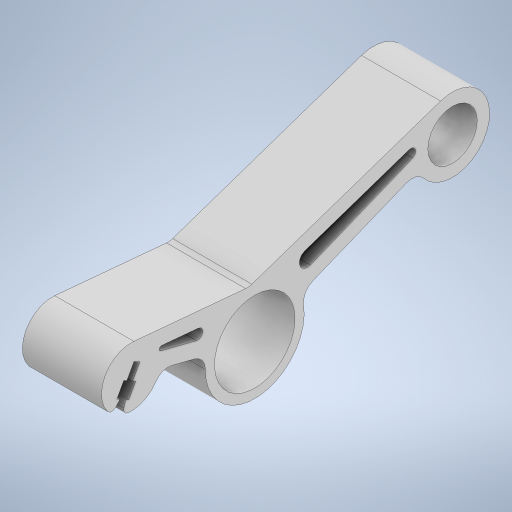
# Autodesk Inventor part: ChargingArm
Saved by Autodesk Inventor 2023 (Build 270158000, 158)
## iProperties
Created: 2023-03-28
Part Number: ChargingArm
Material: Generic
Document SubType Name: Modeling
Designer: ethan
Density: 1 g/cm^3
Appearance: Default
Author: ethan
Autodesk Inventor part; units mm, degrees
ref_plane "YZ Plane" through (0, 0, 0) normal (1, 0, 0) x (0, 1, 0)
ref_plane "XZ Plane" through (0, 0, 0) normal (0, 1, 0) x (-1, 0, 0)
ref_plane "XY Plane" through (0, 0, 0) normal (0, 0, 1) x (1, 0, 0)
sketch "Sketch1" plane through (0, 0, 0) normal (1, 0, 0) x (0, 1, 0)
  circle A0 centre (0, 0) radius 10
  circle A1 centre (0, 0) radius 8.15
  circle A2 centre (0, 0) radius 12.5 construction
  line L0 (41.321287, 101.306893) -> (-14.257578, 0) construction
  line L1 (-14.257578, 0) -> (54.700579, -125.694122) construction
  line L2 (0, 0) -> (-14.257578, 0) construction
  circle A3 centre (16.24172, -40) radius 7.5
  line L3 (23.342454, -37.585547) -> (9.467645, 3.219271)
  line L4 (0, 0) -> (16.24172, -40)
  circle A4 centre (6.301529, 25) radius 6
  line L5 (6.301529, 25) -> (0, 0)
  line L6 (12.276626, 24.45391) -> (9.958495, -0.91015)
  line L7 (6.301529, 25) -> (1.041169, 27.885933) construction
  line L8 (2.571626, 25.477961) -> (5.114134, 24.083094)
  line L9 (5.114134, 24.083094) -> (6.436853, 26.494093)
  line L10 (6.436853, 26.494093) -> (3.894345, 27.88896)
  line L11 (3.894345, 27.88896) -> (2.571626, 25.477961)
  line L12 (2.571626, 25.477961) -> (6.436853, 26.494093) construction
  line L13 (5.114134, 24.083094) -> (3.894345, 27.88896) construction
  line L14 (3.557653, 27.275251) -> (6.100161, 25.880384) construction
  line L15 (6.100161, 25.880384) -> (5.450826, 24.696803) construction
  line L16 (5.450826, 24.696803) -> (2.908318, 26.09167) construction
  line L17 (2.908318, 26.09167) -> (3.557653, 27.275251) construction
  line L18 (3.557653, 27.275251) -> (5.450826, 24.696803) construction
  line L19 (6.100161, 25.880384) -> (2.908318, 26.09167) construction
  line L20 (1.041169, 27.885933) -> (1.720669, 28.875012) construction
  line L21 (1.041169, 27.885933) -> (0.572083, 26.781415) construction
  line L22 (1.720669, 28.875012) -> (3.557653, 27.275251)
  line L23 (0.572083, 26.781415) -> (2.908318, 26.09167)
  circle A5 centre (16.24172, -40) radius 5
  line L24 (6.100161, 25.880384) -> (5.450826, 24.696803)
  line L25 (5.450826, 24.696803) -> (8.081006, 23.253836)
  line L26 (8.081006, 23.253836) -> (8.730341, 24.437418)
  line L27 (8.730341, 24.437418) -> (6.100161, 25.880384)
  line L28 (7.879427, 18.985837) -> (6.064574, 11.785787)
  line L29 (8.750781, 18.837133) -> (8.074972, 11.442697)
  circle A6 centre (8.309301, 18.877482) radius 0.44332
  circle A7 centre (7.056384, 11.53579) radius 1.022833
  line L30 (10.828915, -10.103009) -> (18.023548, -31.261908)
  line L31 (7.742377, -11.093657) -> (16.206515, -31.939079)
  circle A8 centre (9.297434, -10.623756) radius 1.617595
  circle A9 centre (17.10522, -31.574166) radius 0.969965
  point P0 (3.762124, -9.265334)
  point P1 (13.420127, -33.050999)
  point P2 (10.151966, 1.206731)
  point P3 (4.835032, 19.181978)
  point P4 (2.444163, 9.696704)
  point P5 (4.504239, 25.986027)
  point P6 (3.557653, 27.275251)
  point P7 (3.228968, 26.676138)
  point P8 (6.100161, 25.880384)
  point P9 (5.450826, 24.696803)
  point P10 (7.798679, -11.232315)
  dimension "d8" = 15
  dimension "d0" = 20
  dimension "d1" = 16.3
  dimension "d6" = 25
  dimension "d7" = 122.5
  dimension "d9" = 40
  dimension "d10" = 12
  dimension "d11" = 25
  dimension "d14" = 2.9
  dimension "d15" = 2.75
  dimension "d16" = 2.5
  dimension "d17" = 1.35
  dimension "d18" = 1.2
  dimension "d19" = 1.2
  dimension "d20" = 10
  dimension "d24" = 3
  dimension "d25" = 3
  dimension "d26" = 3
  dimension "d30" = 3
  dimension "d31" = 3
  constraints: 64 end point, 14 tangent, 12 point on circle, 11 parallel, 8 centre point, 4 coincident, 4 midpoint, 3 perpendicular, 3 point on line, 1 collinear, 1 horizontal, 12 other
  measures "d0" diameter of A0
  measures "d1" diameter of A1
  measures "d6" diameter of A2
  measures "d7" angle of L1 L0
  measures "d9" vertical distance of L4.end point (0, 0)
  measures "d10" diameter of A4
  measures "d11" vertical distance of point (0, 0) L5.start
  measures "d14" distance of L8.start L8.end
  measures "d15" distance of L9.end L8.end
  measures "d16" distance between parallel lines of L0 L11
  measures "d17" distance between parallel lines of L16 L14
  measures "d18" distance of L7.end L20.end
  measures "d19" distance of L7.end L21.end
  measures "d20" diameter of A5
  measures "d24" distance of L25.end L15.end
  measures "d25" distance between parallel lines of L5 L28
  measures "d26" distance between parallel lines of L6 L29
  measures "d30" distance between parallel lines of L4 L31
  measures "d31" distance between parallel lines of L3 L30
extrude "Extrusion1" add sketch "Sketch1" along normal blind 16 contours A0 L4 A1 L5 | A0 L3 L6 | A0 L5 A4 L6 L3 | L6 L3 A3 L4 A0 | L5 A1 L4 A0 | L5 L25 L26 L27 L9 L10 L11 L22 A4 | A4 L23 L11 L8 L9 L25 L5 | A3
fillet "Fillet1" radius 3 5 edges at (8, 2.4442, 9.6967) (8, 4.835, 19.182) (8, 13.4201, -33.051) (8, 3.7621, -9.2653) (8, 10.152, 1.2067)
fillet "Fillet2" radius 1 2 edges at (8, 1.7207, 28.875) (8, 0.5721, 26.7814)
body "Solid1"
